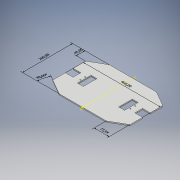
# Autodesk Inventor part: Base_gros_robot
Saved by Autodesk Inventor 2018 (Build 220112000, 112)
## iProperties
Created: 2018-01-30
Part Number: Base_gros_robot
Material: Générique
Document SubType Name: Modeling
Designer: Tristan
Density: 1 g/cm^3
Appearance: Par défaut
Author: Tristan
Autodesk Inventor part; units mm, degrees
ref_plane "XZ Plane" through (0, 0, 0) normal (0, 1, 0) x (-1, 0, 0)
ref_plane "XY Plane" through (0, 0, 0) normal (0, 0, 1) x (1, 0, 0)
sketch "Esquisse1" plane through (0, 0, 0) normal (0, 0, 1) x (1, 0, 0)
  line L0 (0, 0) -> (400, 0)
  line L1 (400, 0) -> (400, -260)
  line L2 (400, -260) -> (0, -260)
  line L3 (0, -260) -> (0, 0)
  dimension "d0" = 400
  dimension "d1" = 260
  constraints: 8 end point, 2 parallel, 1 horizontal, 1 perpendicular
  measures "d0" distance of L0.start L0.end
  measures "d1" distance of L0.end L1.end
extrude "Extrusion1" add sketch "Esquisse1" along normal blind 6
chamfer "Chanfrein1" distance 45 angle 60 2 edges at (400, -260, 3) (400, 0, 3) measured on face at (400, -86.6667, 2)
chamfer "Chanfrein2" distance 45 angle 60 2 edges at (0, -260, 3) (0, 0, 3) measured on face at (0, -173.3333, 2)
sketch "Esquisse4" plane through (0, 0, 6) normal (0, 0, 1) x (1, 0, 0)
  line L0 (0, -150) -> (40, -150)
  line L1 (40, -150) -> (40, -110)
  line L2 (40, -110) -> (0, -110)
  line L3 (0, -110) -> (0, -150)
  line L4 (322.0577, 0) -> (77.9423, 0) projected
  line L5 (77.9423, -260) -> (322.0577, -260) projected
  line L6 (0, -45) -> (0, -215) projected
  line L7 (77.9423, -95) -> (107.9423, -95)
  line L8 (107.9423, -95) -> (107.9423, -165)
  line L9 (107.9423, -165) -> (77.9423, -165)
  line L10 (77.9423, -165) -> (77.9423, -95)
  point P0 (0, 0)
  dimension "d77" = 40
  dimension "d81" = 40
  dimension "d82" = 110
  dimension "d83" = 110
  dimension "d91" = 0
  dimension "d92" = 70
  dimension "d93" = 95
  dimension "d94" = 95
  dimension "d95" = 30
  constraints: 16 end point, 4 parallel, 2 horizontal, 2 perpendicular
  measures "d77" distance of L0.start L0.end
  measures "d81" distance of L0.end L1.end
  measures "d82" distance between parallel lines of L2 L4
  measures "d83" distance between parallel lines of L5 L0
  measures "d91" distance between parallel lines of L6 L3
  measures "d92" distance of L9.end L7.start
  measures "d93" distance between parallel lines of L4 L7
  measures "d94" distance between parallel lines of L5 L9
  measures "d95" distance of L7.start L7.end
extrude "Extrusion4" cut sketch "Esquisse4" against normal blind 40
ref_plane "Plan de construction1" through (200, -260, 6) normal (1, 0, 0) x (0, 1, 0)
hole "Perçage1" at (70.4423, -117.5, 6) direction (0, 0, -1) diameter 5 end through all
hole "Perçage2" at (70.4423, -142.5, 6) direction (0, 0, -1) diameter 5 end through all
mirror "Symétrie1" about plane through (200, -260, 6) normal (1, 0, 0) of "Extrusion4", "Perçage2", "Perçage1"
equation "\"d86\" = d81"
